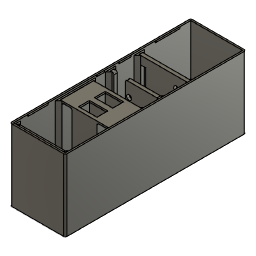
RFID case v12 (Autodesk Fusion 360 design; units mm, degrees)
Autodesk Fusion 360 part; units mm, degrees
note: some values were not read from the file. Chosen so that the rebuilt part matches the saved one: which bodies a step acts on.
(part 1 of 2)
sketch "Sketch4" plane through (0, 0, 0) normal (0, 1, 0) x (1, 0, 0) in component "Main Case"
  line L0 (0, 0) -> (2, 0)
  line L1 (2, 0) -> (2, 4.6)
  line L2 (2, 4.6) -> (0, 4.6) construction
  line L3 (0, 4.6) -> (0, 0)
  line L4 (0, 4.6) -> (0, 54.6)
  line L5 (0, 54.6) -> (0, 95.2)
  line L6 (0, 95.2) -> (0, 115.2)
  line L7 (0, 115.2) -> (0, 119.8)
  line L8 (0, 119.8) -> (0, 149.8)
  line L9 (0, 149.8) -> (0, 154.4)
  line L10 (0, 154.4) -> (0, 214.4)
  line L11 (0, 54.6) -> (2, 54.6) construction
  line L12 (2, 54.6) -> (4, 54.6)
  circle A0 centre (0, 54.6) radius 4 construction
  line L13 (4, 54.6) -> (0, 50.6)
  line L14 (0, 95.2) -> (2, 95.2) construction
  line L15 (2, 95.2) -> (4, 95.2)
  circle A1 centre (0, 95.2) radius 4 construction
  line L16 (4, 95.2) -> (0, 99.2)
  line L17 (2, 95.2) -> (2, 54.6)
  line L18 (2, 4.6) -> (4, 4.6)
  circle A2 centre (0, 4.6) radius 4 construction
  line L19 (4, 4.6) -> (0, 8.6)
  line L20 (0, 115.2) -> (2, 115.2) construction
  line L21 (2, 115.2) -> (4, 115.2)
  circle A3 centre (0, 115.2) radius 4 construction
  line L22 (4, 115.2) -> (0, 111.2)
  line L23 (0, 119.8) -> (2, 119.8) construction
  line L24 (2, 119.8) -> (4, 119.8)
  circle A4 centre (0, 119.8) radius 4 construction
  line L25 (4, 119.8) -> (0, 123.8)
  line L26 (2, 119.8) -> (2, 115.2)
  line L27 (0, 149.8) -> (2, 149.8) construction
  line L28 (2, 149.8) -> (4, 149.8)
  line L29 (0, 154.4) -> (2, 154.4) construction
  line L30 (2, 154.4) -> (4, 154.4)
  circle A5 centre (0, 154.4) radius 4 construction
  circle A6 centre (0, 149.8) radius 4 construction
  line L31 (4, 154.4) -> (0, 158.4)
  line L32 (4, 149.8) -> (0, 145.8)
  line L33 (2, 149.8) -> (2, 154.4)
  line L34 (0, 0) -> (62.7, 0)
  line L35 (62.7, 0) -> (0, 0)
  line L36 (0, 0) -> (0, 214.4)
  line L37 (0, 214.4) -> (62.7, 214.4)
  line L38 (62.7, 214.4) -> (62.7, 0)
  line L39 (64.7, -2) -> (-2, -2)
  line L40 (-2, -2) -> (-2, 216.4)
  line L41 (-2, 216.4) -> (64.7, 216.4)
  line L42 (64.7, 216.4) -> (64.7, -2)
  line L43 (31.35, 0) -> (31.35, 214.4) construction
  line L44 (58.7, 154.4) -> (62.7, 158.4)
  line L45 (60.7, 154.4) -> (58.7, 154.4)
  line L46 (60.7, 149.8) -> (60.7, 154.4)
  line L47 (60.7, 149.8) -> (58.7, 149.8)
  line L48 (58.7, 149.8) -> (62.7, 145.8)
  line L49 (58.7, 119.8) -> (62.7, 123.8)
  line L50 (60.7, 119.8) -> (58.7, 119.8)
  line L51 (60.7, 119.8) -> (60.7, 115.2)
  line L52 (60.7, 115.2) -> (58.7, 115.2)
  line L53 (58.7, 115.2) -> (62.7, 111.2)
  line L54 (58.7, 95.2) -> (62.7, 99.2)
  line L55 (60.7, 95.2) -> (60.7, 54.6)
  line L56 (60.7, 95.2) -> (58.7, 95.2)
  line L57 (60.7, 54.6) -> (58.7, 54.6)
  line L58 (58.7, 54.6) -> (62.7, 50.6)
  line L59 (58.7, 4.6) -> (62.7, 8.6)
  line L60 (60.7, 0) -> (60.7, 4.6)
  line L61 (60.7, 4.6) -> (58.7, 4.6)
  line L62 (58.7, 54.6) -> (4, 54.6)
  line L63 (4, 95.2) -> (58.7, 95.2) construction
  line L64 (31.35, 95.2) -> (31.35, 54.6) construction
  circle A7 centre (31.35, 74.9) radius 12.5
  line L65 (58.7, 4.6) -> (58.7, 0)
  line L66 (4, 4.6) -> (4, 0)
  dimension "d121" = 2
  dimension "d122" = 4.6
  dimension "d146" = 50
  dimension "d147" = 40.6
  dimension "d148" = 20
  dimension "d149" = 4.6
  dimension "d150" = 30
  dimension "d151" = 4.6
  dimension "d152" = 60
  dimension "d153" = 2
  dimension "d154" = 2
  dimension "d155" = 2
  dimension "d156" = 2
  dimension "d157" = 2
  dimension "d158" = 2
  dimension "d159" = 2
  dimension "d160" = 2
  dimension "d161" = 2
  dimension "d162" = 2
  dimension "d163" = 2
  dimension "d164" = 2
  dimension "d165" = 2
  dimension "d166" = 62.7
  dimension "d512" = 25
  constraint horizontal L0
  constraint vertical L1
  constraint horizontal L2
  constraint vertical L3
  constraint coincident L0.start L3.end
  constraint collinear L3 L4
  constraint collinear L4 L5
  constraint collinear L5 L6
  constraint parallel L6 L7
  constraint collinear L7 L8
  constraint parallel L8 L9
  constraint parallel L9 L10
  constraint perpendicular L5 L11
  constraint perpendicular L5 L12
  constraint coincident L4.end L5.start
  constraint coincident L12.end A0
  constraint coincident A0 L13.end
  constraint coincident L4 L13.end
  constraint perpendicular L5 L14
  constraint perpendicular L5 L15
  constraint coincident L5.end L6.start
  constraint coincident L15.end A1
  constraint coincident A1 L16.end
  constraint coincident L6 L16.end
  constraint perpendicular L1 L18
  constraint coincident L2.end L3.start
  constraint coincident L18.end A2
  constraint coincident A2 L19.end
  constraint coincident L4 L19.end
  constraint perpendicular L7 L20
  constraint perpendicular L7 L21
  constraint coincident L6.end L7.start
  constraint coincident L21.end A3
  constraint coincident A3 L22.end
  constraint coincident L6 L22.end
  constraint perpendicular L8 L23
  constraint perpendicular L8 L24
  constraint coincident L7.end L8.start
  constraint coincident L24.end A4
  constraint coincident A4 L25.end
  constraint coincident L8 L25.end
  constraint perpendicular L9 L27
  constraint perpendicular L9 L28
  constraint perpendicular L9 L29
  constraint perpendicular L9 L30
  constraint coincident L9.end L10.start
  constraint coincident L30.end A5
  constraint coincident L8.end L9.start
  constraint coincident L28.end A6
  constraint coincident A5 L31.end
  constraint coincident L10 L31.end
  constraint coincident A6 L32.end
  constraint coincident L8 L32.end
  constraint perpendicular L3 L34
  constraint horizontal L35
  constraint vertical L36
  constraint horizontal L37
  constraint vertical L38
  constraint midpoint L35 L43.start
  constraint midpoint L37 L43.end
  constraint symmetric L0.end L43 L60.start
  constraint symmetric L1.end L43 L60.end
  constraint symmetric L11.end L43 L55.end
  constraint symmetric L12.end L43 L57.end
  constraint symmetric L13.end L43 L58.end
  constraint symmetric L14.end L43 L55.start
  constraint symmetric L15.end L43 L54.start
  constraint symmetric L16.end L43 L54.end
  constraint symmetric L18.end L43 L59.start
  constraint symmetric L19.end L43 L59.end
  constraint symmetric L20.end L43 L51.end
  constraint symmetric L21.end L43 L52.end
  constraint symmetric L22.end L43 L53.end
  constraint symmetric L23.end L43 L50.start
  constraint symmetric L24.end L43 L49.start
  constraint symmetric L25.end L43 L49.end
  constraint symmetric L27.end L43 L46.start
  constraint symmetric L28.end L43 L47.end
  constraint symmetric L29.end L43 L45.start
  constraint symmetric L30.end L43 L44.start
  constraint symmetric L31.end L43 L44.end
  constraint symmetric L32.end L43 L48.end
  constraint midpoint L63 L64.start
  constraint midpoint L62 L64.end
  constraint midpoint L64 A7.centre
  constraint coincident L35 L65.end
  constraint perpendicular L35 L65
  constraint coincident L34 L66.end
  constraint perpendicular L34 L66
  measures "d121" distance of L0.start L0.end
  measures "d122" distance of L0.start L2.end
  measures "d146" distance of L2.end L4.end
  measures "d147" distance of L4.end L5.end
  measures "d148" distance of L5.end L6.end
  measures "d149" distance of L6.end L7.end
  measures "d150" distance of L7.end L8.end
  measures "d151" distance of L8.end L9.end
  measures "d152" distance of L9.end L10.end
  measures "d153" distance of L4.end L11.end
  measures "d154" distance of L11.end L12.end
  measures "d155" distance of L5.end L14.end
  measures "d156" distance of L14.end L15.end
  measures "d157" distance of L1.end L18.end
  measures "d158" distance of L6.end L20.end
  measures "d159" distance of L20.end L21.end
  measures "d160" distance of L7.end L23.end
  measures "d161" distance of L23.end L24.end
  measures "d162" distance of L8.end L27.end
  measures "d163" distance of L27.end L28.end
  measures "d164" distance of L9.end L29.end
  measures "d165" distance of L29.end L30.end
  measures "d166" distance of L0.start L34.end
  measures "d512" diameter of A7
extrude "Extrude7" add sketch "Sketch4" along normal blind 84.4 contours L0 L1 L3 L4 L18 L19 L34 L35 L36 | L4 L5 L6 L12 L13 L15 L16 L17 L36 | L34 L35 L38 L59 L60 L61 | L38 L54 L55 L56 L57 L58 | L6 L7 L8 L21 L22 L24 L25 L26 L36 | L38 L49 L50 L51 L52 L53 | L38 L44 L45 L46 L47 L48 | L8 L9 L10 L28 L30 L31 L32 L33 L36 makes body 1 at (62.7, 28.1333, -83) makes body 2 at (0, 28.1333, -115.4) makes body 3 at (0, 56.2667, -150) makes body 4 at (62.7, 28.1333, -5.7333) makes body 5 at (62.7, 28.1333, -119.6) makes body 6 at (0, 28.1333, -66.8) makes body 7 at (62.7, 56.2667, -154.2) makes body 8 at (0, 56.2667, -2.8667) in component "Main Case"
extrude "Extrude8" add sketch "Sketch4" along normal blind 2 contours L1 L18 L34 L35 L66 | L4 L13 L19 L34 L35 L36 L38 L58 L59 L62 L65 L66 | L34 L35 L60 L61 L65 | L6 L8 L10 L12 L15 L16 L17 L21 L22 L24 L25 L26 L28 L30 L31 L32 L33 L36 L37 L38 L44 L45 L46 L47 L48 L49 L50 L51 L52 L53 L54 L55 L56 L57 L62 | A7 bodies 1 2 3 4 5 6 7 8 in component "Main Case"
extrude "Extrude9" add sketch "Sketch4" along normal blind 86.6 contours L39 L40 L41 L42 bodies 1 in component "Main Case"
fillet "Fillet1" radius 2 4 edges at (-2, 43.3, -216.4) (64.7, 43.3, -216.4) (64.7, 43.3, 2) (-2, 43.3, 2) on bodies 1 in component "Main Case"
sketch "Sketch5" plane through (0, 2, 0) normal (0, 1, 0) x (-1, 0, 0) in component "Main Case"
  line L0 (-60.7, 0) -> (-60.7, -4.6)
  line L1 (-60.7, -4.6) -> (-58.7, -4.6)
  line L2 (-58.7, -4.6) -> (-62.7, -8.6)
  line L3 (-62.7, -8.6) -> (-62.7, -50.6)
  line L4 (-62.7, -50.6) -> (-58.7, -54.6)
  line L5 (-58.7, -54.6) -> (-60.7, -54.6)
  line L6 (-60.7, -54.6) -> (-60.7, -95.2)
  line L7 (-60.7, -95.2) -> (-58.7, -95.2)
  line L8 (-58.7, -95.2) -> (-62.7, -99.2)
  line L9 (-62.7, -99.2) -> (-62.7, -111.2)
  line L10 (-62.7, -111.2) -> (-58.7, -115.2)
  line L11 (-58.7, -115.2) -> (-60.7, -115.2)
  line L12 (-60.7, -115.2) -> (-60.7, -119.8)
  line L13 (-60.7, -119.8) -> (-58.7, -119.8)
  line L14 (-58.7, -119.8) -> (-62.7, -123.8)
  line L15 (-62.7, -123.8) -> (-62.7, -145.8)
  line L16 (-62.7, -145.8) -> (-58.7, -149.8)
  line L17 (-58.7, -149.8) -> (-60.7, -149.8)
  line L18 (-60.7, -149.8) -> (-60.7, -154.4)
  line L19 (-60.7, -154.4) -> (-58.7, -154.4)
  line L20 (-58.7, -154.4) -> (-62.7, -158.4)
  line L21 (-62.7, -158.4) -> (-62.7, -214.4)
  line L22 (-62.7, -214.4) -> (0, -214.4)
  line L23 (0, -214.4) -> (0, -158.4)
  line L24 (0, -158.4) -> (-4, -154.4)
  line L25 (-4, -154.4) -> (-2, -154.4)
  line L26 (-2, -154.4) -> (-2, -149.8)
  line L27 (-2, -149.8) -> (-4, -149.8)
  line L28 (-4, -149.8) -> (0, -145.8)
  line L29 (0, -145.8) -> (0, -123.8)
  line L30 (0, -123.8) -> (-4, -119.8)
  line L31 (-4, -119.8) -> (-2, -119.8)
  line L32 (-2, -119.8) -> (-2, -115.2)
  line L33 (-2, -115.2) -> (-4, -115.2)
  line L34 (-4, -115.2) -> (0, -111.2)
  line L35 (0, -111.2) -> (0, -99.2)
  line L36 (0, -99.2) -> (-4, -95.2)
  line L37 (-4, -95.2) -> (-2, -95.2)
  line L38 (-2, -95.2) -> (-2, -54.6)
  line L39 (-2, -54.6) -> (-4, -54.6)
  line L40 (-4, -54.6) -> (0, -50.6)
  line L41 (0, -50.6) -> (0, -8.6)
  line L42 (0, -8.6) -> (-4, -4.6)
  line L43 (-4, -4.6) -> (-2, -4.6)
  line L44 (-2, -4.6) -> (-2, 0)
  line L45 (-2, 0) -> (-60.7, 0)
  line L46 (-2, 0) -> (-2, -2) construction
  line L47 (-2, -2) -> (-60.7, -2)
  line L48 (-4, -4.6) -> (-58.7, -4.6)
  line L49 (-4, -154.4) -> (-58.7, -154.4) construction
  line L50 (-31.35, -154.4) -> (-31.35, -214.4) construction
  circle A0 centre (-31.35, -184.4) radius 3.25
  line L51 (0, -8.6) -> (0, -25.8) construction
  line L52 (0, -25.8) -> (-2, -25.8) construction
  line L53 (-2, -25.8) -> (-60.7, -25.8)
  line L54 (-58.7, -4.6) -> (-58.7, 0)
  line L55 (-4, -4.6) -> (-4, 0)
  dimension "d176" = 2
  dimension "d180" = 6.5
  dimension "d507" = 17.2
  constraint coincident L44.end L45.start
  constraint coincident L44 L46.end
  constraint coincident L0 L47.end
  constraint perpendicular L0 L47
  constraint coincident L42.end L43.start
  constraint coincident L1.end L2.start
  constraint coincident L24.end L25.start
  constraint coincident L19.end L20.start
  constraint midpoint L49 L50.start
  constraint midpoint L22 L50.end
  constraint midpoint L50 A0.centre
  constraint coincident L41.end L42.start
  constraint parallel L41 L51
  constraint coincident L38 L52.end
  constraint perpendicular L38 L52
  constraint coincident L6 L53.end
  constraint perpendicular L6 L53
  constraint coincident L45 L54.end
  constraint perpendicular L45 L54
  constraint coincident L45 L55.end
  constraint perpendicular L45 L55
  measures "d176" distance of L44.end L46.end
  measures "d180" diameter of A0
  measures "d507" distance of L41.end L51.end
extrude "Extrude10" cut sketch "Sketch5" against normal blind 2 contours L47 L48 L54 L55 bodies 1 in component "Main Case"
extrude "Extrude11" cut sketch "Sketch5" against normal blind 2 contours A0 bodies 1 in component "Main Case"
sketch "Sketch6" plane through (0, 0, 0) normal (1, 0, 0) x (0, 0, -1) in component "Main Case"
  line L0 (0, 84.4) -> (8.6, 84.4)
  line L1 (8.6, 84.4) -> (8.6, 2)
  line L2 (8.6, 2) -> (50.6, 2)
  line L3 (50.6, 2) -> (50.6, 84.4)
  line L4 (50.6, 84.4) -> (99.2, 84.4)
  line L5 (99.2, 84.4) -> (99.2, 2)
  line L6 (99.2, 2) -> (111.2, 2)
  line L7 (111.2, 2) -> (111.2, 84.4)
  line L8 (111.2, 84.4) -> (123.8, 84.4)
  line L9 (123.8, 84.4) -> (123.8, 2)
  line L10 (123.8, 2) -> (145.8, 2)
  line L11 (145.8, 2) -> (145.8, 84.4)
  line L12 (145.8, 84.4) -> (158.4, 84.4)
  line L13 (158.4, 84.4) -> (158.4, 2)
  line L14 (158.4, 2) -> (214.4, 2)
  line L15 (214.4, 2) -> (214.4, 86.6)
  line L16 (214.4, 86.6) -> (0, 86.6)
  line L17 (0, 86.6) -> (0, 84.4)
  line L18 (8.6, 84.4) -> (50.6, 84.4) construction
  line L19 (17.1, 86.6) -> (42.1, 86.6)
  line L20 (42.1, 86.6) -> (42.1, 84.6)
  line L21 (42.1, 84.6) -> (17.1, 84.6)
  line L22 (17.1, 84.6) -> (17.1, 86.6)
  line L23 (29.6, 84.4) -> (29.6, 86.6) construction
  line L24 (99.2, 84.4) -> (111.2, 84.4) construction
  line L25 (100.2, 86.6) -> (110.2, 86.6)
  line L26 (110.2, 86.6) -> (110.2, 84.6)
  line L27 (110.2, 84.6) -> (100.2, 84.6)
  line L28 (100.2, 84.6) -> (100.2, 86.6)
  line L29 (105.2, 86.6) -> (105.2, 84.4) construction
  line L30 (123.8, 84.4) -> (145.8, 84.4) construction
  line L31 (127.3, 86.6) -> (142.3, 86.6)
  line L32 (142.3, 86.6) -> (142.3, 84.6)
  line L33 (142.3, 84.6) -> (127.3, 84.6)
  line L34 (127.3, 84.6) -> (127.3, 86.6)
  line L35 (134.8, 84.4) -> (134.8, 86.6) construction
  line L36 (158.4, 84.4) -> (214.4, 84.4) construction
  line L37 (171.4, 86.6) -> (201.4, 86.6)
  line L38 (201.4, 86.6) -> (201.4, 84.6)
  line L39 (201.4, 84.6) -> (171.4, 84.6)
  line L40 (171.4, 84.6) -> (171.4, 86.6)
  line L41 (186.4, 84.4) -> (186.4, 86.6) construction
  dimension "d183" = 25
  dimension "d184" = 2
  dimension "d185" = 10
  dimension "d186" = 2
  dimension "d187" = 15
  dimension "d188" = 2
  dimension "d189" = 30
  dimension "d190" = 2
  constraint coincident L0.end L1.start
  constraint coincident L3.end L4.start
  constraint horizontal L19
  constraint vertical L20
  constraint horizontal L21
  constraint vertical L22
  constraint coincident L16 L19.start
  constraint midpoint L18 L23.start
  constraint midpoint L19 L23.end
  constraint perpendicular L19 L23
  constraint coincident L4.end L5.start
  constraint coincident L7.end L8.start
  constraint horizontal L25
  constraint vertical L26
  constraint horizontal L27
  constraint vertical L28
  constraint coincident L16 L25.start
  constraint midpoint L25 L29.start
  constraint midpoint L24 L29.end
  constraint perpendicular L16 L29
  constraint coincident L8.end L9.start
  constraint coincident L11.end L12.start
  constraint horizontal L31
  constraint vertical L32
  constraint horizontal L33
  constraint vertical L34
  constraint coincident L16 L31.start
  constraint midpoint L30 L35.start
  constraint midpoint L31 L35.end
  constraint perpendicular L16 L35
  constraint coincident L12.end L13.start
  constraint coincident L15 L36.end
  constraint perpendicular L15 L36
  constraint horizontal L37
  constraint vertical L38
  constraint horizontal L39
  constraint vertical L40
  constraint coincident L16 L37.start
  constraint midpoint L36 L41.start
  constraint midpoint L37 L41.end
  constraint perpendicular L16 L41
  measures "d183" distance of L19.start L19.end
  measures "d184" distance of L19.start L21.end
  measures "d185" distance of L25.start L25.end
  measures "d186" distance of L25.start L27.end
  measures "d187" distance of L31.start L31.end
  measures "d188" distance of L31.start L33.end
  measures "d189" distance of L37.start L37.end
  measures "d190" distance of L37.start L39.end
extrude "Extrude12" add sketch "Sketch6" along normal blind 4 draft -45 contours L16 L19 L20 L21 L22 | L16 L25 L26 L27 L28 | L16 L31 L32 L33 L34 | L16 L37 L38 L39 L40 bodies 1 in component "Main Case"
ref_plane "WorkPlane1" through (31.35, 43.3, -107.2) normal (-1, 0, 0) x (0, 0, 1) in component "Main Case"
mirror "Mirror1" about plane through (31.35, 43.3, -107.2) normal (-1, 0, 0) of "Extrude12" in component "Main Case"
sketch "Sketch1" plane through (0, 86.6, 0) normal (0, 1, 0) x (-1, 0, 0) in component "Case Lid"
  arc A0 (2, 0) -> (0, 2) centre (0, 0) ccw
  line L0 (0, 2) -> (-62.7, 2)
  arc A1 (-62.7, 2) -> (-64.7, 0) centre (-62.7, 0) ccw
  line L1 (-64.7, 0) -> (-64.7, -214.4)
  arc A2 (-64.7, -214.4) -> (-62.7, -216.4) centre (-62.7, -214.4) ccw
  line L2 (-62.7, -216.4) -> (0, -216.4)
  arc A3 (0, -216.4) -> (2, -214.4) centre (0, -214.4) ccw
  line L3 (2, -214.4) -> (2, 0)
  line L4 (0, -214.4) -> (-62.7, -214.4)
  line L5 (-62.7, -214.4) -> (-62.7, -201.4)
  line L6 (-62.7, -201.4) -> (-62.7, -171.4)
  line L7 (-62.7, -171.4) -> (-62.7, -142.3)
  line L8 (-62.7, -142.3) -> (-62.7, -127.3)
  line L9 (-62.7, -127.3) -> (-62.7, -110.2)
  line L10 (-62.7, -110.2) -> (-62.7, -100.2)
  line L11 (-62.7, -100.2) -> (-62.7, -42.1)
  line L12 (-62.7, -42.1) -> (-62.7, -17.1)
  line L13 (-62.7, -17.1) -> (-62.7, 0)
  line L14 (-62.7, 0) -> (0, 0)
  line L15 (0, 0) -> (0, -17.1)
  line L16 (0, -17.1) -> (0, -42.1)
  line L17 (0, -42.1) -> (0, -100.2)
  line L18 (0, -100.2) -> (0, -110.2)
  line L19 (0, -110.2) -> (0, -127.3)
  line L20 (0, -127.3) -> (0, -142.3)
  line L21 (0, -142.3) -> (0, -171.4)
  line L22 (0, -171.4) -> (0, -201.4)
  line L23 (0, -201.4) -> (0, -214.4)
extrude "Extrude1" add sketch "Sketch1" along normal blind 2 separate body contours A0 L0 A1 L1 A2 L2 A3 L3 | L4 L5 L6 L7 L8 L9 L10 L11 L12 L13 L14 L15 L16 L17 L18 L19 L20 L21 L22 L23 makes body 9 in component "Case Lid"
sketch "Sketch2" plane through (0, 86.6, 0) normal (0, -1, 0) x (1, 0, 0) in component "Case Lid"
  line L0 (-2, 0) -> (-2, -214.4)
  arc A0 (-2, -214.4) -> (0, -216.4) centre (0, -214.4) ccw
  line L1 (0, -216.4) -> (62.7, -216.4)
  arc A1 (62.7, -216.4) -> (64.7, -214.4) centre (62.7, -214.4) ccw
  line L2 (64.7, -214.4) -> (64.7, 0)
  arc A2 (64.7, 0) -> (62.7, 2) centre (62.7, 0) ccw
  line L3 (62.7, 2) -> (0, 2)
  arc A3 (0, 2) -> (-2, 0) centre (0, 0) ccw
  line L4 (0.2, -0.2) -> (0.2, -214.2)
  line L5 (0.2, -214.2) -> (62.5, -214.2)
  line L6 (62.5, -214.2) -> (62.5, -0.2)
  line L7 (62.5, -0.2) -> (0.2, -0.2)
extrude "Extrude2" add sketch "Sketch2" along normal blind 2 contours L4 L5 L6 L7 bodies 9 in component "Case Lid"
extrude "Extrude3" cut sketch "Sketch6" along normal blind 4 draft -45 from surface at 0.2 contours L16 L19 L20 L21 L22 | L16 L25 L26 L27 L28 | L16 L31 L32 L33 L34 | L16 L37 L38 L39 L40 bodies 9 in component "Case Lid"
mirror "Mirror2" about plane through (31.35, 43.3, -107.2) normal (-1, 0, 0) of "Extrude3" in component "Case Lid"
shell "Shell1" thickness 2 removed faces 1 at (41.7333, 84.6, -80.8333) on bodies 9 in component "Case Lid"
chamfer "Chamfer1" distance 0.6 angle 45 8 edges at (62.5, 84.6, -186.4) (62.5, 84.6, -134.8) (62.5, 84.6, -105.2) (62.5, 84.6, -29.6) (0.2, 84.6, -29.6) (0.2, 84.6, -105.2) (0.2, 84.6, -134.8) (0.2, 84.6, -186.4) on bodies 9 in component "Case Lid"
sketch "Sketch1 (2)" plane through (0, 2, 0) normal (0, 1, 0) x (-1, 0, 0) in component "UnoShelfV2"
  circle A0 centre (-31.35, -184.4) radius 3.25
  line L0 (-4, -4.6) -> (-58.7, -4.6)
  line L1 (-58.7, -4.6) -> (-62.7, -8.6)
  line L2 (-62.7, -8.6) -> (-62.7, -50.6)
  line L3 (-62.7, -50.6) -> (-58.7, -54.6)
  line L4 (-58.7, -54.6) -> (-60.7, -54.6)
  line L5 (-60.7, -54.6) -> (-60.7, -95.2)
  line L6 (-60.7, -95.2) -> (-58.7, -95.2)
  line L7 (-58.7, -95.2) -> (-62.7, -99.2)
  line L8 (-62.7, -99.2) -> (-62.7, -111.2)
  line L9 (-62.7, -111.2) -> (-58.7, -115.2)
  line L10 (-58.7, -115.2) -> (-60.7, -115.2)
  line L11 (-60.7, -115.2) -> (-60.7, -119.8)
  line L12 (-60.7, -119.8) -> (-58.7, -119.8)
  line L13 (-58.7, -119.8) -> (-62.7, -123.8)
  line L14 (-62.7, -123.8) -> (-62.7, -145.8)
  line L15 (-62.7, -145.8) -> (-58.7, -149.8)
  line L16 (-58.7, -149.8) -> (-60.7, -149.8)
  line L17 (-60.7, -149.8) -> (-60.7, -154.4)
  line L18 (-60.7, -154.4) -> (-58.7, -154.4)
  line L19 (-58.7, -154.4) -> (-62.7, -158.4)
  line L20 (-62.7, -158.4) -> (-62.7, -214.4)
  line L21 (-62.7, -214.4) -> (0, -214.4)
  line L22 (0, -214.4) -> (0, -158.4)
  line L23 (0, -158.4) -> (-4, -154.4)
  line L24 (-4, -154.4) -> (-2, -154.4)
  line L25 (-2, -154.4) -> (-2, -149.8)
  line L26 (-2, -149.8) -> (-4, -149.8)
  line L27 (-4, -149.8) -> (0, -145.8)
  line L28 (0, -145.8) -> (0, -123.8)
  line L29 (0, -123.8) -> (-4, -119.8)
  line L30 (-4, -119.8) -> (-2, -119.8)
  line L31 (-2, -119.8) -> (-2, -115.2)
  line L32 (-2, -115.2) -> (-4, -115.2)
  line L33 (-4, -115.2) -> (0, -111.2)
  line L34 (0, -111.2) -> (0, -99.2)
  line L35 (0, -99.2) -> (-4, -95.2)
  line L36 (-4, -95.2) -> (-2, -95.2)
  line L37 (-2, -95.2) -> (-2, -54.6)
  line L38 (-2, -54.6) -> (-4, -54.6)
  line L39 (-4, -54.6) -> (0, -50.6)
  line L40 (0, -50.6) -> (0, -8.6)
  line L41 (0, -8.6) -> (-4, -4.6)
  line L42 (-2, 0) -> (-60.5, 0) construction
  line L43 (-2.1, 0) -> (-60.4, 0)
  line L44 (-60.4, 0) -> (-60.4, -4.2)
  line L45 (-60.4, -4.2) -> (-2.1, -4.2)
  line L46 (-2.1, -4.2) -> (-2.1, 0)
  line L47 (-31.25, 0) -> (-31.25, -4.2) construction
  dimension "d377" = 58.3
  dimension "d378" = 4.2
  constraint horizontal L42
  constraint horizontal L43
  constraint vertical L44
  constraint horizontal L45
  constraint vertical L46
  constraint coincident L42 L43.start
  constraint midpoint L42 L47.start
  constraint midpoint L45 L47.end
  constraint perpendicular L42 L47
  measures "d377" distance of L43.start L43.end
  measures "d378" distance of L43.start L45.end
extrude "Extrude1'" add sketch "Sketch1 (2)" along normal blind 82.4 separate body contours L43 L44 L45 L46 makes body 10 in component "UnoShelfV2"
sketch "Sketch2 (2)" plane through (0, 0, -4.2) normal (0, 0, -1) x (-1, 0, 0) in component "UnoShelfV2"
  line L0 (-60.4, 2) -> (-2.1, 2)
  line L1 (-2.1, 2) -> (-2.1, 84.4)
  line L2 (-2.1, 84.4) -> (-60.4, 84.4)
  line L3 (-60.4, 84.4) -> (-60.4, 2)
  line L4 (-11.8, 2) -> (-11.8, 70.2) construction
  line L5 (-2.1, 70.2) -> (-11.8, 70.2) construction
  line L6 (-2.1, 70.2) -> (-39.7, 70.2) construction
  line L7 (-39.7, 2) -> (-39.7, 70.2) construction
  circle A0 centre (-11.8, 70.2) radius 1.7
  circle A1 centre (-39.7, 70.2) radius 1.7
  circle A2 centre (-39.7, 70.2) radius 3
  circle A3 centre (-11.8, 70.2) radius 3
  line L8 (-2.1, 18.1) -> (-6.7, 18.1) construction
  line L9 (-6.7, 18.1) -> (-6.7, 2) construction
  circle A4 centre (-6.7, 18.1) radius 3
  circle A5 centre (-6.7, 18.1) radius 1.7
  line L10 (-55.7, 2) -> (-55.7, 19.4) construction
  line L11 (-55.7, 19.4) -> (-60.4, 19.4) construction
  circle A6 centre (-55.7, 19.4) radius 3
  circle A7 centre (-55.7, 19.4) radius 1.7
  dimension "d381" = 68.2
  dimension "d382" = 9.7
  dimension "d383" = 37.6
  dimension "d384" = 68.2
  dimension "d385" = 3.4
  dimension "d386" = 3.4
  dimension "d387" = 6
  dimension "d388" = 6
  dimension "d520" = 4.6
  dimension "d521" = 16.1
  dimension "d522" = 6
  dimension "d523" = 3.4
  dimension "d524" = 17.4
  dimension "d525" = 4.7
  dimension "d526" = 6
  dimension "d527" = 3.4
  constraint coincident L0 L4.start
  constraint perpendicular L0 L4
  constraint coincident L1 L5.start
  constraint perpendicular L4 L5
  constraint perpendicular L1 L6
  constraint coincident L0 L7.start
  constraint perpendicular L0 L7
  constraint coincident L4.end L5.end
  constraint coincident L6.end L7.end
  constraint concentric A1 A2
  constraint concentric A0 A3
  constraint coincident L1 L8.start
  constraint perpendicular L1 L8
  constraint coincident L0 L9.end
  constraint perpendicular L0 L9
  constraint coincident L8.end L9.start
  constraint concentric A4 A5
  constraint coincident L0 L10.start
  constraint perpendicular L0 L10
  constraint coincident L3 L11.end
  constraint perpendicular L3 L11
  constraint coincident L10.end L11.start
  constraint concentric A6 A7
  measures "d381" distance of L4.start L4.end
  measures "d382" distance of L4.end L5.start
  measures "d383" distance of L5.start L6.end
  measures "d384" vertical distance of L6.end L7.start
  measures "d385" diameter of A0
  measures "d386" diameter of A1
  measures "d387" diameter of A2
  measures "d388" diameter of A3
  measures "d520" distance of L8.start L8.end
  measures "d521" distance of L8.end L9.end
  measures "d522" diameter of A4
  measures "d523" diameter of A5
  measures "d524" distance of L10.start L10.end
  measures "d525" distance of L10.end L11.end
  measures "d526" diameter of A6
  measures "d527" diameter of A7
extrude "Extrude2'" cut sketch "Sketch2 (2)" against normal up to surface (4.2 mm away) contours A0 | A1 | A5 | A7 bodies 10 in component "UnoShelfV2"
extrude "Extrude3'" cut sketch "Sketch2 (2)" along normal blind 3.2 from surface at -4.2 contours A2 | A3 | A4 | A6 bodies 10 in component "UnoShelfV2"
fillet "Fillet1'" radius 2 4 edges at (60.4, 84.4, -2.1) (2.1, 84.4, -2.1) (60.4, 2, -2.1) (2.1, 2, -2.1) on bodies 10 in component "UnoShelfV2"
sketch "Sketch1 (3)" plane through (0, 2, 0) normal (0, 1, 0) x (-1, 0, 0) in component "BatteryShelf"
  circle A0 centre (-31.35, -184.4) radius 3.25
  line L0 (-4, -4.6) -> (-58.7, -4.6)
  line L1 (-58.7, -4.6) -> (-62.7, -8.6)
  line L2 (-62.7, -8.6) -> (-62.7, -50.6)
  line L3 (-62.7, -50.6) -> (-58.7, -54.6)
  line L4 (-58.7, -54.6) -> (-60.7, -54.6)
  line L5 (-60.7, -54.6) -> (-60.7, -95.2)
  line L6 (-60.7, -115.2) -> (-60.7, -119.8)
  line L7 (-60.7, -119.8) -> (-58.7, -119.8)
  line L8 (-58.7, -119.8) -> (-62.7, -123.8)
  line L9 (-62.7, -123.8) -> (-62.7, -145.8)
  line L10 (-62.7, -145.8) -> (-58.7, -149.8)
  line L11 (-58.7, -149.8) -> (-60.7, -149.8)
  line L12 (-60.7, -149.8) -> (-60.7, -154.4)
  line L13 (-60.7, -154.4) -> (-58.7, -154.4)
  line L14 (-58.7, -154.4) -> (-62.7, -158.4)
  line L15 (-62.7, -158.4) -> (-62.7, -214.4)
  line L16 (-62.7, -214.4) -> (0, -214.4)
  line L17 (0, -214.4) -> (0, -158.4)
  line L18 (0, -158.4) -> (-4, -154.4)
  line L19 (-4, -154.4) -> (-2, -154.4)
  line L20 (-2, -154.4) -> (-2, -149.8)
  line L21 (-2, -149.8) -> (-4, -149.8)
  line L22 (-4, -149.8) -> (0, -145.8)
  line L23 (0, -145.8) -> (0, -123.8)
  line L24 (0, -123.8) -> (-4, -119.8)
  line L25 (-4, -119.8) -> (-2, -119.8)
  line L26 (-2, -119.8) -> (-2, -115.2)
  line L27 (-2, -95.2) -> (-2, -54.6)
  line L28 (-2, -54.6) -> (-4, -54.6)
  line L29 (-4, -54.6) -> (0, -50.6)
  line L30 (0, -50.6) -> (0, -8.6)
  line L31 (0, -8.6) -> (-4, -4.6)
  line L32 (-2.2, -54.6) -> (-60.5, -54.6)
  line L33 (-60.5, -54.6) -> (-60.5, -94.8)
  line L34 (-60.5, -94.8) -> (-2.2, -94.8)
  line L35 (-2.2, -94.8) -> (-2.2, -54.6)
  line L36 (-4, -54.6) -> (-58.7, -54.6) construction
  line L37 (-31.35, -54.6) -> (-31.35, -94.8) construction
  line L38 (-18.3, -73.7) -> (-44.4, -73.7)
  line L39 (-44.4, -73.7) -> (-44.4, -56.6)
  line L40 (-44.4, -56.6) -> (-18.3, -56.6)
  line L41 (-18.3, -56.6) -> (-18.3, -73.7)
  line L42 (-31.35, -54.6) -> (-31.35, -56.6) construction
  line L43 (-18.3, -73.7) -> (-18.3, -75.7) construction
  line L44 (-18.3, -75.7) -> (-44.4, -75.7)
  line L45 (-44.4, -75.7) -> (-44.4, -92.8)
  line L46 (-44.4, -92.8) -> (-18.3, -92.8)
  line L47 (-18.3, -92.8) -> (-18.3, -75.7)
  line L48 (-42.4, -71.7) -> (-42.4, -58.6)
  line L49 (-42.4, -58.6) -> (-20.3, -58.6)
  line L50 (-20.3, -58.6) -> (-20.3, -71.7)
  line L51 (-20.3, -71.7) -> (-42.4, -71.7)
  line L52 (-20.3, -90.8) -> (-20.3, -77.7)
  line L53 (-20.3, -77.7) -> (-42.4, -77.7)
  line L54 (-42.4, -77.7) -> (-42.4, -90.8)
  line L55 (-42.4, -90.8) -> (-20.3, -90.8)
  line L56 (-2.2, -54.6) -> (-4.2, -54.6) construction
  line L57 (-4.2, -54.6) -> (-4.2, -94.8)
  line L58 (-60.5, -54.6) -> (-58.5, -54.6) construction
  line L59 (-58.5, -54.6) -> (-58.5, -94.8)
  line L60 (-44.4, -75.7) -> (-44.4, -73.7) construction
  line L61 (-18.3, -75.7) -> (-18.3, -73.7) construction
  line L62 (-18.3, -56.6) -> (-16.3, -56.6) construction
  line L63 (-16.3, -56.6) -> (-16.3, -54.6)
  line L64 (-16.3, -56.6) -> (-16.3, -94.8)
  line L65 (-44.4, -56.6) -> (-46.4, -56.6) construction
  line L66 (-46.4, -56.6) -> (-46.4, -54.6)
  line L67 (-46.4, -56.6) -> (-46.4, -94.8)
  dimension "d248" = 58.3
  dimension "d249" = 40.2
  dimension "d258" = 26.1
  dimension "d259" = 17.1
  dimension "d260" = 2
  dimension "d261" = 2
  dimension "d262" = 26.1
  dimension "d263" = 17.1
  dimension "d264" = 2
  dimension "d266" = 2
  dimension "d267" = 2
  dimension "d268" = 2
  dimension "d269" = 2
  constraint horizontal L32
  constraint vertical L33
  constraint horizontal L34
  constraint vertical L35
  constraint coincident L28 L32.start
  constraint coincident L28.end L29.start
  constraint coincident L3.end L4.start
  constraint midpoint L36 L37.start
  constraint midpoint L34 L37.end
  constraint perpendicular L36 L37
  constraint horizontal L38
  constraint vertical L39
  constraint horizontal L40
  constraint vertical L41
  constraint midpoint L40 L42.end
  constraint perpendicular L36 L42
  constraint perpendicular L38 L43
  constraint horizontal L44
  constraint vertical L45
  constraint horizontal L46
  constraint vertical L47
  constraint perpendicular L35 L56
  constraint coincident L34 L57.end
  constraint perpendicular L34 L57
  constraint perpendicular L33 L58
  constraint coincident L34 L59.end
  constraint perpendicular L34 L59
  constraint perpendicular L41 L62
  constraint coincident L36 L63.end
  constraint perpendicular L36 L63
  constraint coincident L34 L64.end
  constraint perpendicular L34 L64
  constraint perpendicular L39 L65
  constraint coincident L36 L66.end
  constraint perpendicular L36 L66
  constraint coincident L34 L67.end
  constraint perpendicular L34 L67
  measures "d248" distance of L32.start L32.end
  measures "d249" distance of L32.start L34.end
  measures "d258" distance of L38.start L38.end
  measures "d259" distance of L38.start L40.end
  measures "d260" distance of L37.start L42.end
  measures "d261" distance of L38.start L43.end
  measures "d262" distance of L43.end L44.end
  measures "d263" distance of L43.end L46.end
  measures "d266" distance of L32.start L56.end
  measures "d267" distance of L32.end L58.end
  measures "d268" distance of L40.end L62.end
  measures "d269" distance of L39.end L65.end
extrude "Extrude1''" add sketch "Sketch1 (3)" along normal blind 82.4 separate body contours L28 L32 L34 L35 L57 | L4 L32 L33 L34 L59 makes body 11 at (2.2, 56.9333, -81.4) makes body 12 at (58.5, 29.4667, -68) in component "BatteryShelf"
sketch "Sketch3" plane through (4.2, 0, 0) normal (1, 0, 0) x (0, 0, -1) in component "BatteryShelf"
  line L0 (54.6, 2) -> (94.8, 2)
  line L1 (94.8, 2) -> (94.8, 84.4)
  line L2 (94.8, 84.4) -> (54.6, 84.4)
  line L3 (54.6, 84.4) -> (54.6, 2)
  line L4 (54.6, 84.4) -> (54.6, 82.4) construction
  line L5 (54.6, 82.4) -> (94.8, 82.4)
  dimension "d288" = 2
  constraint coincident L2.end L3.start
  constraint coincident L3 L4.end
  constraint coincident L1 L5.end
  constraint perpendicular L1 L5
  measures "d288" distance of L2.end L4.end
extrude "Extrude7'" add sketch "Sketch3" along normal blind 54.3 contours L1 L2 L3 L5 bodies 11 12 in component "BatteryShelf"
extrude "Extrude8'" cut sketch "Sketch1 (3)" along normal up to surface (2 mm away) from surface at 80.4 contours L48 L49 L50 L51 | L52 L53 L54 L55 bodies 11 in component "BatteryShelf"
extrude "Extrude9'" add sketch "Sketch1 (3)" against normal blind 47 from surface at 80.4 contours L32 L34 L63 L64 L66 L67 bodies 11 in component "BatteryShelf"
sketch "Sketch4 (2)" plane through (0, 0, -54.6) normal (0, 0, 1) x (1, 0, 0) in component "BatteryShelf"
  line L0 (2.2, 2) -> (4.2, 2)
  line L1 (4.2, 2) -> (4.2, 82.4)
  line L2 (4.2, 82.4) -> (16.3, 82.4)
  line L3 (16.3, 82.4) -> (16.3, 35.4)
  line L4 (16.3, 35.4) -> (46.4, 35.4)
  line L5 (46.4, 35.4) -> (46.4, 82.4)
  line L6 (46.4, 82.4) -> (58.5, 82.4)
  line L7 (58.5, 82.4) -> (58.5, 2)
  line L8 (58.5, 2) -> (60.5, 2)
  line L9 (60.5, 2) -> (60.5, 84.4)
  line L10 (60.5, 84.4) -> (2.2, 84.4)
  line L11 (2.2, 84.4) -> (2.2, 2)
  line L12 (24.85, 35.4) -> (37.85, 35.4)
  line L13 (37.85, 35.4) -> (37.85, 37.4)
  line L14 (37.85, 37.4) -> (24.85, 37.4)
  line L15 (24.85, 37.4) -> (24.85, 35.4)
  line L16 (31.35, 35.4) -> (31.35, 37.4) construction
  dimension "d297" = 13
  dimension "d298" = 2
  constraint horizontal L12
  constraint vertical L13
  constraint horizontal L14
  constraint vertical L15
  constraint coincident L4 L12.start
  constraint midpoint L4 L16.start
  constraint midpoint L14 L16.end
  constraint perpendicular L4 L16
  measures "d297" distance of L12.start L12.end
  measures "d298" distance of L12.start L14.end
extrude "Extrude10'" add sketch "Sketch4 (2)" along normal blind 4 draft -45 from surface at -19.1 contours L4 L12 L13 L14 L15 bodies 11 in component "BatteryShelf"
extrude "Extrude11'" add sketch "Sketch4 (2)" against normal blind 4 draft -45 from surface at -21.1 contours L4 L12 L13 L14 L15 bodies 11 in component "BatteryShelf"
sketch "Sketch1 (4)" plane through (0, 2, 0) normal (0, 1, 0) x (-1, 0, 0) in component "ConverterShelf"
  circle A0 centre (-31.35, -184.4) radius 3.25
  line L0 (-4, -4.6) -> (-58.7, -4.6)
  line L1 (-58.7, -4.6) -> (-62.7, -8.6)
  line L2 (-62.7, -8.6) -> (-62.7, -50.6)
  line L3 (-62.7, -50.6) -> (-58.7, -54.6)
  line L4 (-58.7, -54.6) -> (-60.7, -54.6)
  line L5 (-60.7, -54.6) -> (-60.7, -95.2)
  line L6 (-60.7, -95.2) -> (-58.7, -95.2)
  line L7 (-58.7, -95.2) -> (-62.7, -99.2)
  line L8 (-62.7, -99.2) -> (-62.7, -111.2)
  line L9 (-62.7, -111.2) -> (-58.7, -115.2)
  line L10 (-58.7, -115.2) -> (-60.7, -115.2)
  line L11 (-60.7, -115.2) -> (-60.7, -119.8)
  line L12 (-60.7, -119.8) -> (-58.7, -119.8)
  line L13 (-58.7, -119.8) -> (-62.7, -123.8)
  line L14 (-62.7, -123.8) -> (-62.7, -145.8)
  line L15 (-62.7, -145.8) -> (-58.7, -149.8)
  line L16 (-58.7, -149.8) -> (-60.7, -149.8)
  line L17 (-60.7, -149.8) -> (-60.7, -154.4)
  line L18 (-60.7, -154.4) -> (-58.7, -154.4)
  line L19 (-58.7, -154.4) -> (-62.7, -158.4)
  line L20 (-62.7, -158.4) -> (-62.7, -214.4)
  line L21 (-62.7, -214.4) -> (0, -214.4)
  line L22 (0, -214.4) -> (0, -158.4)
  line L23 (0, -158.4) -> (-4, -154.4)
  line L24 (-4, -154.4) -> (-2, -154.4)
  line L25 (-2, -154.4) -> (-2, -149.8)
  line L26 (-2, -149.8) -> (-4, -149.8)
  line L27 (-4, -149.8) -> (0, -145.8)
  line L28 (0, -145.8) -> (0, -123.8)
  line L29 (0, -123.8) -> (-4, -119.8)
  line L30 (-4, -119.8) -> (-2, -119.8)
  line L31 (-2, -119.8) -> (-2, -115.2)
  line L32 (-2, -115.2) -> (-4, -115.2)
  line L33 (-4, -115.2) -> (0, -111.2)
  line L34 (0, -111.2) -> (0, -99.2)
  line L35 (0, -99.2) -> (-4, -95.2)
  line L36 (-4, -95.2) -> (-2, -95.2)
  line L37 (-2, -95.2) -> (-2, -54.6)
  line L38 (-2, -54.6) -> (-4, -54.6)
  line L39 (-4, -54.6) -> (0, -50.6)
  line L40 (0, -50.6) -> (0, -8.6)
  line L41 (0, -8.6) -> (-4, -4.6)
  line L42 (-4, -115.2) -> (-58.7, -115.2)
  line L43 (-2.2, -115.2) -> (-60.5, -115.2)
  line L44 (-60.5, -115.2) -> (-60.5, -119.4)
  line L45 (-60.5, -119.4) -> (-2.2, -119.4)
  line L46 (-2.2, -119.4) -> (-2.2, -115.2)
  line L47 (-31.35, -115.2) -> (-31.35, -119.4) construction
  line L48 (-2.2, -115.2) -> (-2.2023, -117.2) construction
  line L49 (-60.5, -118.0847) -> (-58.4, -118.0847) construction
  line L50 (-2.2, -104.7885) -> (-4.3, -104.7885) construction
  line L51 (-4.3, -119.4) -> (-4.3, -106.2)
  line L52 (-4.3, -106.2) -> (-18, -106.2)
  line L53 (-18, -106.2) -> (-18, -119.4)
  dimension "d309" = 58.3
  dimension "d310" = 4.2
  dimension "d417" = 2.1
  dimension "d418" = 2.1
  dimension "d420" = 13.7
  dimension "d489" = 13.2
  constraint coincident L32.end L33.start
  constraint coincident L9.end L10.start
  constraint horizontal L43
  constraint vertical L44
  constraint horizontal L45
  constraint vertical L46
  constraint coincident L42 L43.start
  constraint midpoint L42 L47.start
  constraint midpoint L45 L47.end
  constraint perpendicular L42 L47
  constraint coincident L44 L49.start
  constraint perpendicular L44 L49
  constraint coincident L46 L50.start
  constraint perpendicular L46 L50
  constraint coincident L45 L51.start
  constraint coincident L45 L53.end
  constraint perpendicular L45 L51
  constraint coincident L50.end L51
  constraint perpendicular L45 L53
  constraint perpendicular L52 L53
  measures "d309" distance of L43.start L43.end
  measures "d310" distance of L43.start L45.end
  measures "d417" distance of L49.start L49.end
  measures "d418" distance of L50.start L50.end
  measures "d420" distance of L51.end L52.end
  measures "d489" distance of L51.end L51.start
extrude "Extrude7''" add sketch "Sketch1 (4)" along normal blind 82.4 separate body contours L32 L42 L43 L45 L46 L51 | L10 L42 L43 L44 L45 L53 | L42 L43 L45 L51 L53 makes body 13 in component "ConverterShelf"
extrude "Extrude8''" add sketch "Sketch1 (4)" along normal blind 20.6 contours L42 L43 L45 L51 L53 | L42 L43 L51 L52 L53 bodies 13 in component "ConverterShelf"
sketch "Sketch12" plane through (0, 2, 0) normal (0, -1, 0) x (1, 0, 0) in component "ConverterShelf"
  line L0 (4.3, -115.2) -> (2.2, -115.2)
  line L1 (2.2, -115.2) -> (2.2, -119.4)
  line L2 (2.2, -119.4) -> (60.5, -119.4)
  line L3 (60.5, -119.4) -> (60.5, -115.2)
  line L4 (60.5, -115.2) -> (18, -115.2)
  line L5 (18, -115.2) -> (18, -106.2)
  line L6 (18, -106.2) -> (4.3, -106.2)
  line L7 (4.3, -106.2) -> (4.3, -115.2)
  circle A0 centre (4.3, -106.2) radius 4 construction
  circle A1 centre (18, -106.2) radius 4 construction
  line L8 (4.3, -110.2) -> (8.3, -106.2)
  line L9 (14, -106.2) -> (18, -110.2)
  line L10 (4.3, -85.6031) -> (6.3, -85.6031) construction
  line L11 (6.3, -119.4) -> (6.3, -108.2)
  line L12 (16, -108.2) -> (16, -119.4)
  line L13 (6.3, -117.4) -> (16, -117.4)
  line L14 (9.3137, -117.4) -> (9.3137, -119.4) construction
  dimension "d490" = 8
  dimension "d491" = 8
  dimension "d493" = 2
  constraint coincident L6.end L7.start
  constraint coincident L5.end L6.start
  constraint coincident A0 L8.start
  constraint coincident L7 L8.start
  constraint coincident L6 L8.end
  constraint coincident A0 L8.end
  constraint coincident A1 L9.start
  constraint coincident L6 L9.start
  constraint coincident A1 L9.end
  constraint coincident L5 L9.end
  constraint coincident L7 L10.start
  constraint perpendicular L7 L10
  constraint coincident L2 L11.start
  constraint midpoint L8 L11.end
  constraint coincident L10.end L11
  constraint perpendicular L2 L11
  constraint midpoint L9 L12.start
  constraint coincident L2 L12.end
  constraint perpendicular L2 L12
  constraint coincident L11 L13.start
  constraint coincident L12 L13.end
  constraint perpendicular L12 L13
  constraint coincident L13 L14.start
  constraint coincident L2 L14.end
  constraint perpendicular L2 L14
  measures "d490" diameter of A0
  measures "d491" diameter of A1
  measures "d493" distance of L14.start L14.end
extrude "Extrude17" cut sketch "Sketch12" against normal blind 16.6 contours L6 L8 L9 L11 L12 L13 bodies 13 in component "ConverterShelf"
sketch "Sketch13" plane through (0, 0, -117.4) normal (0, 0, 1) x (1, 0, 0) in component "ConverterShelf"
  line L0 (6.3, 2) -> (16, 2)
  line L1 (16, 2) -> (16, 18.6)
  line L2 (16, 18.6) -> (6.3, 18.6)
  line L3 (6.3, 18.6) -> (6.3, 2)
  line L4 (9.2223, 2) -> (9.2223, 4) construction
  line L5 (6.3, 4) -> (16, 4)
  dimension "d501" = 2
  constraint coincident L0 L4.start
  constraint perpendicular L0 L4
  constraint coincident L3 L5.start
  constraint coincident L1 L5.end
  constraint perpendicular L1 L5
  constraint coincident L4.end L5
  measures "d501" distance of L4.start L4.end
extrude "Extrude18" cut sketch "Sketch13" against normal blind 2 contours L1 L2 L3 L5 bodies 13 in component "ConverterShelf"
sketch "Sketch14" plane through (6.3, 0, 0) normal (1, 0, 0) x (0, 0, -1) in component "ConverterShelf"
  line L0 (108.2, 2) -> (117.4, 2)
  line L1 (119.4, 4) -> (119.4, 18.6)
  line L2 (119.4, 18.6) -> (108.2, 18.6)
  line L3 (108.2, 18.6) -> (108.2, 2)
  line L4 (84.875, 2) -> (92.125, 2)
  line L5 (119.4, 14.95) -> (117.4, 14.95)
  line L6 (117.4, 14.95) -> (117.4, 7.65)
  line L7 (117.4, 7.65) -> (119.4, 7.65)
  line L8 (119.4, 7.65) -> (119.4, 14.95)
  line L9 (117.4, 2) -> (117.4, 4)
  line L10 (117.4, 4) -> (119.4, 4)
  line L11 (119.4, 11.3) -> (117.4, 11.3) construction
  dimension "d498" = 7.25
  dimension "d499" = 2
  dimension "d500" = 7.3
  constraint horizontal L4
  constraint coincident L0 L4.start
  constraint horizontal L5
  constraint vertical L6
  constraint horizontal L7
  constraint vertical L8
  constraint coincident L1 L5.start
  constraint midpoint L1 L11.start
  constraint midpoint L6 L11.end
  constraint perpendicular L8 L11
  measures "d498" distance of L4.start L4.end
  measures "d499" distance of L5.start L5.end
  measures "d500" distance of L5.start L7.end
extrude "Extrude19" add sketch "Sketch14" along normal blind 4 draft -45 contours L1 L5 L6 L7 L8 bodies 13 in component "ConverterShelf"
sketch "Sketch10" plane through (0, 0, -119.4) normal (0, 0, -1) x (-1, 0, 0) in component "ConverterShelf"
  line L0 (-60.5, 2) -> (-2.2, 2)
  line L1 (-2.2, 2) -> (-2.2, 84.4)
  line L2 (-2.2, 84.4) -> (-60.5, 84.4)
  line L3 (-60.5, 84.4) -> (-60.5, 2)
  line L4 (-60.5, 2) -> (-2.2, 2) construction
  line L5 (-60.5, 19.7828) -> (-58.3, 19.7828) construction
  line L6 (-58.3174, 2.0486) -> (-58.2503, 70.4086) construction
  line L7 (-58.2503, 70.4086) -> (-22.1103, 70.3731) construction
  line L8 (-22.1103, 70.3731) -> (-22.1103, 2.0069) construction
  line L9 (-22.1103, 2.0069) -> (-22.1101, 4.2069) construction
  line L10 (-22.1101, 4.2069) -> (-58.3153, 4.2424) construction
  line L11 (-24.6128, 4.2093) -> (-24.6103, 6.7093) construction
  line L12 (-24.6103, 6.7093) -> (-22.1103, 6.7069) construction
  line L13 (-55.8153, 4.24) -> (-55.8128, 6.74) construction
  line L14 (-55.8128, 6.74) -> (-58.3128, 6.7424) construction
  line L15 (-58.2527, 67.9086) -> (-55.7527, 67.9061) construction
  line L16 (-55.7527, 67.9061) -> (-55.7503, 70.4061) construction
  line L17 (-24.6078, 70.3755) -> (-24.6103, 67.8755) construction
  line L18 (-24.6103, 67.8755) -> (-22.1103, 67.8731) construction
  circle A0 centre (-55.7527, 67.9061) radius 1.7
  circle A1 centre (-55.7527, 67.9061) radius 3
  circle A2 centre (-24.6103, 67.8755) radius 1.7
  circle A3 centre (-24.6103, 67.8755) radius 3
  circle A4 centre (-24.6103, 6.7093) radius 1.7
  circle A5 centre (-24.6103, 6.7093) radius 3
  circle A6 centre (-55.8128, 6.74) radius 1.7
  circle A7 centre (-55.8128, 6.74) radius 3
  line L19 (-22.1103, 14.2766) -> (-20.1103, 14.2766) construction
  line L20 (-2.2, 23.4814) -> (-6.2, 23.4814) construction
  line L21 (-6.2, 23.4814) -> (-6.2, 24.6)
  line L22 (-6.2, 24.6) -> (-20.1103, 24.6)
  line L23 (-20.1103, 24.6) -> (-20.1103, 84.4)
  line L24 (-20.1103, 84.4) -> (-6.2, 84.4)
  line L25 (-6.2, 84.4) -> (-6.2, 23.4814)
  line L26 (-16, 4) -> (-16, 18.6)
  line L27 (-16, 18.6) -> (-6.3, 18.6)
  line L28 (-6.3, 18.6) -> (-6.3, 14.95)
  line L29 (-6.3, 14.95) -> (-6.3, 7.65)
  line L30 (-6.3, 7.65) -> (-6.3, 4)
  line L31 (-6.3, 4) -> (-16, 4)
  dimension "d433" = 2.2
  dimension "d434" = 68.36
  dimension "d435" = 36.14
  dimension "d436" = 2.2
  dimension "d437" = 2.5
  dimension "d438" = 2.5
  dimension "d439" = 2.5
  dimension "d440" = 2.5
  dimension "d441" = 2.5
  dimension "d442" = 2.5
  dimension "d443" = 2.5
  dimension "d444" = 2.5
  dimension "d445" = 3.4
  dimension "d446" = 6
  dimension "d447" = 3.4
  dimension "d448" = 6
  dimension "d449" = 3.4
  dimension "d450" = 6
  dimension "d451" = 3.4
  dimension "d452" = 6
  dimension "d458" = 2
  dimension "d459" = 4
  constraint coincident L3 L5.start
  constraint perpendicular L3 L5
  constraint coincident L5.end L6
  constraint perpendicular L6 L7
  constraint perpendicular L4 L8
  constraint coincident L6 L10.end
  constraint perpendicular L6 L10
  constraint coincident L10 L11.start
  constraint perpendicular L10 L11
  constraint perpendicular L11 L12
  constraint coincident L10 L13.start
  constraint perpendicular L10 L13
  constraint perpendicular L6 L14
  constraint coincident L6 L15.start
  constraint perpendicular L6 L15
  constraint perpendicular L7 L16
  constraint coincident L7 L17.start
  constraint perpendicular L7 L17
  constraint perpendicular L17 L18
  constraint coincident L8 L18.end
  constraint coincident L7 L16.end
  constraint coincident L6 L14.end
  constraint coincident L8 L12.end
  constraint coincident L15.end L16.start
  constraint concentric A0 A1
  constraint coincident L17.end L18.start
  constraint concentric A2 A3
  constraint coincident L11.end L12.start
  constraint concentric A4 A5
  constraint coincident L13.end L14.start
  constraint concentric A6 A7
  constraint coincident L8 L19.start
  constraint perpendicular L8 L19
  constraint coincident L1 L20.start
  constraint perpendicular L1 L20
  constraint perpendicular L21 L22
  constraint perpendicular L22 L23
  constraint coincident L19.end L23
  constraint perpendicular L23 L24
  constraint perpendicular L24 L25
  constraint coincident L2 L23.end
  constraint coincident L2 L24.end
  measures "d433" distance of L5.start L5.end
  measures "d434" distance of L6.start L6.end
  measures "d435" distance of L6.end L7.end
  measures "d436" distance of L8.end L9.end
  measures "d437" distance of L11.start L11.end
  measures "d438" distance of L11.end L12.end
  measures "d439" distance of L13.start L13.end
  measures "d440" distance of L13.end L14.end
  measures "d441" distance of L15.start L15.end
  measures "d442" distance of L15.end L16.end
  measures "d443" distance of L17.start L17.end
  measures "d444" distance of L17.end L18.end
  measures "d445" diameter of A0
  measures "d446" diameter of A1
  measures "d447" diameter of A2
  measures "d448" diameter of A3
  measures "d449" diameter of A4
  measures "d450" diameter of A5
  measures "d451" diameter of A6
  measures "d452" diameter of A7
  measures "d458" distance of L19.start L19.end
  measures "d459" distance of L20.start L20.end
extrude "Extrude11''" cut sketch "Sketch10" against normal up to surface (3.2 mm away) from surface at -1 contours A1 | A3 | A5 | A7 bodies 13 in component "ConverterShelf"
extrude "Extrude12'" cut sketch "Sketch10" against normal blind 4.2 contours A0 | A2 | A4 | A6 bodies 13 in component "ConverterShelf"
extrude "Extrude16" cut sketch "Sketch10" against normal blind 4.2 contours L2 L22 L23 L24 L25 bodies 13 in component "ConverterShelf"
fillet "Fillet3" radius 2 2 edges at (20.1103, 24.6, -117.3) (6.2, 24.6, -117.3) on bodies 13 in component "ConverterShelf"
fillet "Fillet3" radius 2 2 edges at (6.2, 84.4, -117.3) (20.1103, 84.4, -117.3) on bodies 13 in component "ConverterShelf"
fillet "Fillet4" radius 2 8 edges at (4.3, 2, -110.7) (4.3, 22.6, -110.7) (18, 22.6, -110.7) (18, 2, -110.7) (60.5, 2, -117.3) (60.5, 84.4, -117.3) (2.2, 84.4, -117.3) (2.2, 2, -117.3) on bodies 13 in component "ConverterShelf"
fillet "Fillet2" radius 1 4 edges at (60.5, 2, -74.7) (2.2, 2, -74.7) (31.35, 35.4, -56.6) (31.35, 35.4, -92.8) on bodies 11 in component "BatteryShelf"
fillet "Fillet3'" radius 2 4 edges at (58.5, 82.4, -74.7) (4.2, 82.4, -74.7) (16.3, 82.4, -74.7) (46.4, 82.4, -74.7) on bodies 11 in component "BatteryShelf"